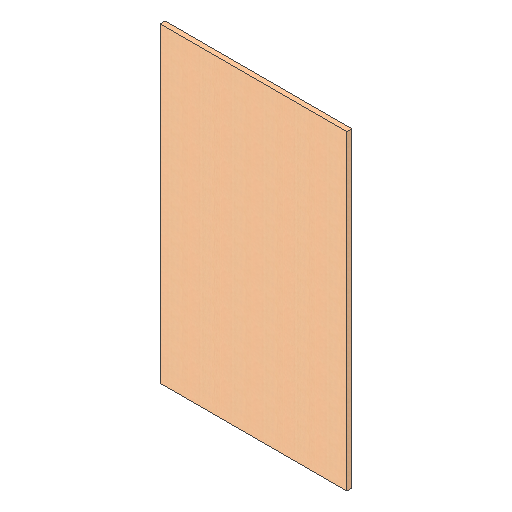
# Autodesk Inventor part: CNCM_WOOD_4mm_Sorting_line_base_plate
Saved by Autodesk Inventor 2026.1 (Build 301233000, 233)
## iProperties
Created: 2018-07-10
Part Number: CNCM_WOOD_4mm_Sorting_line_base_plate
Material: Wood (Birch)
Document SubType Name: Modeling
Designer: Andrzej
Density: 0.55 g/cm^3
Appearance: White Oak
Author: Andrzej
Autodesk Inventor part; units mm, degrees
ref_plane "YZ Plane" through (0, 0, 0) normal (1, 0, 0) x (0, 1, 0)
ref_plane "XZ Plane" through (0, 0, 0) normal (0, 1, 0) x (-1, 0, 0)
ref_plane "XY Plane" through (0, 0, 0) normal (0, 0, 1) x (1, 0, 0)
sketch "Sketch1" plane through (0, 0, 0) normal (0, 0, 1) x (1, 0, 0)
  line L0 (-14.2927, -44.1988) -> (135.7073, -44.1988)
  line L1 (135.7073, -44.1988) -> (135.7073, -294.1988)
  line L2 (135.7073, -294.1988) -> (-14.2927, -294.1988)
  line L3 (-14.2927, -294.1988) -> (-14.2927, -44.1988)
  point P0 (0, 0)
  dimension "d0" = 150
  dimension "d1" = 250
  constraints: 8 end point, 2 parallel, 1 horizontal, 1 perpendicular
  measures "d0" distance of L1.end L2.end
  measures "d1" distance of L0.end L1.end
extrude "Extrusion1" add sketch "Sketch1" along normal blind 4
body "Solid1"
